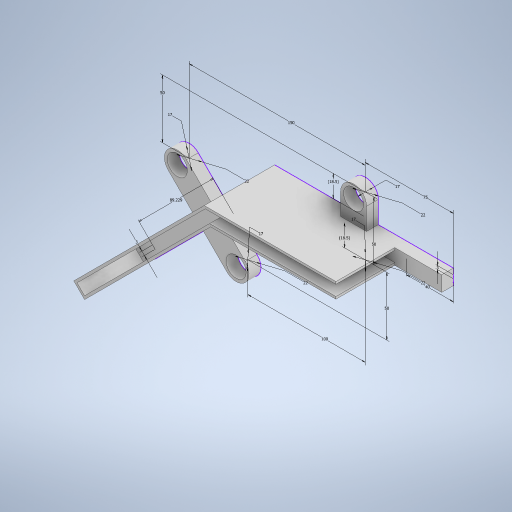
# Autodesk Inventor part: hold_left_sim
Saved by Autodesk Inventor 2024 (Build 280153000, 153)
## iProperties
Created: 2024-02-27
Part Number: hold_left_sim
Material: Generic
Document SubType Name: Modeling
Designer: Administrator
Density: 1 g/cm^3
Appearance: Default
Author: Administrator
Autodesk Inventor part; units mm, degrees
ref_plane "YZ Plane" through (0, 0, 0) normal (1, 0, 0) x (0, 1, 0)
ref_plane "XZ Plane" through (0, 0, 0) normal (0, 1, 0) x (-1, 0, 0)
ref_plane "XY Plane" through (0, 0, 0) normal (0, 0, 1) x (1, 0, 0)
sketch "Sketch1" plane through (0, 0, 0) normal (0, 0, 1) x (1, 0, 0)
  line L0 (-256.066, -104.566) -> (-253.9447, -106.6873)
  line L1 (0, 1.5) -> (0, -1.5)
  line L2 (-263.1371, -104.566) -> (-152.0711, 6.5)
  line L3 (-152.0711, 6.5) -> (0, 6.5)
  line L4 (0, -6.5) -> (-146.6863, -6.5)
  line L5 (-146.6863, -6.5) -> (-253.9447, -113.7584)
  line L6 (-253.9447, -113.7584) -> (-263.1371, -104.566)
  line L7 (0, 1.5) -> (0, 6.5)
  line L8 (0, -1.5) -> (0, -6.5)
  circle A0 centre (-75, 25) radius 11
  circle A1 centre (-175, -75) radius 11
  circle A2 centre (-75, -25) radius 11
  circle A3 centre (-225, -25) radius 11
  line L9 (-232.7782, -32.7782) -> (-212.0637, -53.4926)
  line L10 (-182.7782, -82.7782) -> (-202.8713, -62.685)
  line L11 (-167.2218, -67.2218) -> (-187.315, -47.1287)
  line L12 (-86, 25) -> (-86, 6.5)
  line L13 (-64, 25) -> (-64, 6.5)
  line L14 (-217.2218, -17.2218) -> (-196.5074, -37.9363)
  line L15 (-40, -4.5) -> (-40, -6.5)
  line L16 (-86, -25) -> (-86, -6.5)
  line L17 (-64, -25) -> (-64, -6.5)
  circle A4 centre (-75, 25) radius 8.5
  circle A5 centre (-75, -25) radius 8.5
  circle A6 centre (-175, -75) radius 8.5
  circle A7 centre (-225, -25) radius 8.5
  line L18 (-40, -4.5) -> (-147.5147, -4.5)
  line L19 (-147.5147, -4.5) -> (-253.9447, -110.93)
  line L20 (-253.9447, -110.93) -> (-260.3087, -104.566)
  line L21 (-260.3087, -104.566) -> (-151.2426, 4.5)
  line L22 (-151.2426, 4.5) -> (-40, 4.5)
  line L23 (-40, 4.5) -> (-40, 6.5)
  point P0 (0, 0)
  point P1 (0, 0)
  point P2 (-76.0355, 6.5)
  point P3 (0, -4)
  point P4 (-40, -4.5)
  point P5 (0, -4.5)
  point P6 (0, 4.5)
  dimension "d4" = 3
  dimension "d5" = 3
  dimension "d31" = 22
  dimension "d33" = 22
  dimension "d39" = 75
  dimension "d41" = 22
  dimension "d42" = 50
  dimension "d47" = 22
  dimension "d57" = 18.5
  dimension "d60" = 18.5
  dimension "d62" = 150
  dimension "d63" = 50
  dimension "d64" = 100
  dimension "d65" = 50
  dimension "d66" = 40
  dimension "d70" = 17
  dimension "d71" = 17
  dimension "d72" = 17
  dimension "d73" = 17
  dimension "d78" = 89.2287
  constraints: 48 end point, 11 point on line, 10 perpendicular, 8 centre point, 8 point on circle, 6 tangent, 4 coincident, 3 midpoint, 3 parallel
  measures "d4" distance of L0.start L0.end
  measures "d5" distance of L1.start L1.end
  measures "d31" diameter of A0
  measures "d33" diameter of A1
  measures "d39" horizontal distance of L1.start A0.centre
  measures "d41" diameter of A2
  measures "d42" distance of A2.centre A0.centre
  measures "d47" diameter of A3
  measures "d57" distance from line of L4 A2.centre
  measures "d60" vertical distance of point (-76.036, 6.5) A0.centre
  measures "d62" horizontal distance of A0.centre A3.centre
  measures "d63" vertical distance of A0.centre A3.centre
  measures "d64" horizontal distance of A2.centre A1.centre
  measures "d65" vertical distance of A2.centre A1.centre
  measures "d66" distance from line of point (0, -4) L15
  measures "d70" diameter of A4
  measures "d71" diameter of A5
  measures "d72" diameter of A6
  measures "d73" diameter of A7
  measures "d78" distance between parallel lines of L11 L0
extrude "Extrusion8" add sketch "Sketch1" along normal blind 60 contours L23 L22 L21 L20 L19 L18 L15 L4 L5 L6 L2 L3
extrude "Extrusion9" add sketch "Sketch1" along normal blind 10 contours L1 L8 L4 L15 L18 L19 L20 L21 L22 L23 L3 L7 | L3 L12 A0 L13 | L17 A2 L16 L4 | A0 | A2 | L2 L9 A3 L14 | L11 A1 L10 L5 | A3 | A1
body "Solid5"
